Autodesk Inventor part; units mm, degrees
(part 2 of 2)
  spline S62 degree 3 poles (-7.4168, 223.4534) (-7.297, 223.2633) (-7.1172, 222.9781) (-6.8962, 222.5867) (-6.7374, 222.2894) (-6.5869, 221.9878) (-6.4451, 221.6819) (-6.3131, 221.3718) (-6.1917, 221.0573) (-6.0827, 220.7383) (-5.9867, 220.415) (-5.9243, 220.1411) (-5.8792, 219.921) (-5.8315, 219.7591) (-5.7671, 219.6031) (-5.6832, 219.4564) (-5.5947, 219.3467) (-5.5148, 219.2675) (-5.4472, 219.217) (-5.378, 219.1686) (-5.3017, 219.1325) (-5.2242, 219.099) (-5.1421, 219.0792) (-5.0594, 219.0625) (-4.9468, 219.0585) (-4.8065, 219.061) (-4.6661, 219.0585) (-4.5535, 219.0625) (-4.4708, 219.0792) (-4.3887, 219.099) (-4.3112, 219.1325) (-4.2349, 219.1686) (-4.1657, 219.217) (-4.0981, 219.2675) (-4.0182, 219.3467) (-3.9298, 219.4564) (-3.8458, 219.6031) (-3.7814, 219.7591) (-3.7338, 219.921) (-3.6887, 220.1411) (-3.6262, 220.415) (-3.5303, 220.7383) (-3.4212, 221.0573) (-3.2998, 221.3718) (-3.1678, 221.6819) (-3.0261, 221.9878) (-2.8756, 222.2894) (-2.7167, 222.5867) (-2.4957, 222.9781) (-2.3159, 223.2633) (-2.1961, 223.4534) knots -1.0784 -1.0784 -1.0784 -1.0784 -1.010995 -0.977291 -0.943586 -0.909882 -0.876178 -0.842474 -0.80877 -0.775067 -0.741365 -0.707665 -0.690816 -0.67397 -0.657123 -0.640284 -0.623449 -0.615023 -0.606598 -0.598176 -0.589749 -0.581327 -0.572901 -0.564477 -0.556053 -0.5392 -0.522347 -0.513923 -0.505499 -0.497074 -0.488651 -0.480225 -0.471802 -0.463377 -0.454951 -0.438116 -0.421277 -0.40443 -0.387584 -0.370735 -0.337035 -0.303333 -0.26963 -0.235926 -0.202222 -0.168518 -0.134814 -0.101109 -0.067405 0 0 0 0 construction
  line L30 (-2.1961, 223.4534) -> (-1.1338, 223.4534) construction
  spline S63 degree 3 poles (-1.1338, 223.4534) (-1.014, 223.2633) (-0.8342, 222.9781) (-0.6132, 222.5867) (-0.4544, 222.2894) (-0.3039, 221.9878) (-0.1621, 221.6819) (-0.0301, 221.3718) (0.0913, 221.0573) (0.2003, 220.7383) (0.2963, 220.415) (0.3587, 220.1411) (0.4038, 219.921) (0.4515, 219.7591) (0.5159, 219.6031) (0.5998, 219.4564) (0.6883, 219.3467) (0.7682, 219.2675) (0.8358, 219.217) (0.905, 219.1686) (0.9813, 219.1325) (1.0588, 219.099) (1.1409, 219.0792) (1.2236, 219.0625) (1.3362, 219.0585) (1.4765, 219.061) (1.6169, 219.0585) (1.7295, 219.0625) (1.8122, 219.0792) (1.8943, 219.099) (1.9718, 219.1325) (2.0481, 219.1686) (2.1173, 219.217) (2.1849, 219.2675) (2.2648, 219.3467) (2.3532, 219.4564) (2.4372, 219.6031) (2.5016, 219.7591) (2.5492, 219.921) (2.5943, 220.1411) (2.6568, 220.415) (2.7527, 220.7383) (2.8618, 221.0573) (2.9832, 221.3718) (3.1152, 221.6819) (3.2569, 221.9878) (3.4074, 222.2894) (3.5663, 222.5867) (3.7873, 222.9781) (3.9671, 223.2633) (4.0869, 223.4534) knots -1.0784 -1.0784 -1.0784 -1.0784 -1.010995 -0.977291 -0.943586 -0.909882 -0.876178 -0.842474 -0.80877 -0.775067 -0.741365 -0.707665 -0.690816 -0.67397 -0.657123 -0.640284 -0.623449 -0.615023 -0.606598 -0.598176 -0.589749 -0.581327 -0.572901 -0.564477 -0.556053 -0.5392 -0.522347 -0.513923 -0.505499 -0.497074 -0.488651 -0.480225 -0.471802 -0.463377 -0.454951 -0.438116 -0.421277 -0.40443 -0.387584 -0.370735 -0.337035 -0.303333 -0.26963 -0.235926 -0.202222 -0.168518 -0.134814 -0.101109 -0.067405 0 0 0 0 construction
  line L31 (4.0869, 223.4534) -> (5.1492, 223.4534) construction
  spline S64 degree 3 poles (5.1492, 223.4534) (5.269, 223.2633) (5.4488, 222.9781) (5.6698, 222.5867) (5.8286, 222.2894) (5.9791, 221.9878) (6.1209, 221.6819) (6.2529, 221.3718) (6.3743, 221.0573) (6.4833, 220.7383) (6.5793, 220.415) (6.6417, 220.1411) (6.6868, 219.921) (6.7345, 219.7591) (6.7989, 219.6031) (6.8828, 219.4564) (6.9713, 219.3467) (7.0512, 219.2675) (7.1188, 219.217) (7.188, 219.1686) (7.2643, 219.1325) (7.3418, 219.099) (7.4239, 219.0792) (7.5066, 219.0625) (7.6192, 219.0585) (7.7595, 219.061) (7.8999, 219.0585) (8.0125, 219.0625) (8.0952, 219.0792) (8.1773, 219.099) (8.2548, 219.1325) (8.3311, 219.1686) (8.4003, 219.217) (8.4679, 219.2675) (8.5478, 219.3467) (8.6362, 219.4564) (8.7202, 219.6031) (8.7846, 219.7591) (8.8322, 219.921) (8.8773, 220.1411) (8.9398, 220.415) (9.0357, 220.7383) (9.1448, 221.0573) (9.2662, 221.3718) (9.3982, 221.6819) (9.5399, 221.9878) (9.6904, 222.2894) (9.8493, 222.5867) (10.0703, 222.9781) (10.2501, 223.2633) (10.3699, 223.4534) knots -1.0784 -1.0784 -1.0784 -1.0784 -1.010995 -0.977291 -0.943586 -0.909882 -0.876178 -0.842474 -0.80877 -0.775067 -0.741365 -0.707665 -0.690816 -0.67397 -0.657123 -0.640284 -0.623449 -0.615023 -0.606598 -0.598176 -0.589749 -0.581327 -0.572901 -0.564477 -0.556053 -0.5392 -0.522347 -0.513923 -0.505499 -0.497074 -0.488651 -0.480225 -0.471802 -0.463377 -0.454951 -0.438116 -0.421277 -0.40443 -0.387584 -0.370735 -0.337035 -0.303333 -0.26963 -0.235926 -0.202222 -0.168518 -0.134814 -0.101109 -0.067405 0 0 0 0 construction
  line L32 (10.3699, 223.4534) -> (11.4322, 223.4534) construction
  spline S65 degree 3 poles (11.4322, 223.4534) (11.552, 223.2633) (11.7318, 222.9781) (11.9528, 222.5867) (12.1116, 222.2894) (12.2621, 221.9878) (12.4039, 221.6819) (12.5359, 221.3718) (12.6573, 221.0573) (12.7663, 220.7383) (12.8623, 220.415) (12.9247, 220.1411) (12.9698, 219.921) (13.0175, 219.7591) (13.0819, 219.6031) (13.1658, 219.4564) (13.2543, 219.3467) (13.3342, 219.2675) (13.4018, 219.217) (13.471, 219.1686) (13.5473, 219.1325) (13.6248, 219.099) (13.7069, 219.0792) (13.7896, 219.0625) (13.9022, 219.0585) (14.0425, 219.061) (14.1829, 219.0585) (14.2955, 219.0625) (14.3782, 219.0792) (14.4603, 219.099) (14.5378, 219.1325) (14.6141, 219.1686) (14.6833, 219.217) (14.7509, 219.2675) (14.8308, 219.3467) (14.9192, 219.4564) (15.0032, 219.6031) (15.0676, 219.7591) (15.1152, 219.921) (15.1603, 220.1411) (15.2228, 220.415) (15.3187, 220.7383) (15.4278, 221.0573) (15.5492, 221.3718) (15.6812, 221.6819) (15.8229, 221.9878) (15.9734, 222.2894) (16.1323, 222.5867) (16.3533, 222.9781) (16.5331, 223.2633) (16.6529, 223.4534) knots -1.0784 -1.0784 -1.0784 -1.0784 -1.010995 -0.977291 -0.943586 -0.909882 -0.876178 -0.842474 -0.80877 -0.775067 -0.741365 -0.707665 -0.690816 -0.67397 -0.657123 -0.640284 -0.623449 -0.615023 -0.606598 -0.598176 -0.589749 -0.581327 -0.572901 -0.564477 -0.556053 -0.5392 -0.522347 -0.513923 -0.505499 -0.497074 -0.488651 -0.480225 -0.471802 -0.463377 -0.454951 -0.438116 -0.421277 -0.40443 -0.387584 -0.370735 -0.337035 -0.303333 -0.26963 -0.235926 -0.202222 -0.168518 -0.134814 -0.101109 -0.067405 0 0 0 0 construction
  line L33 (16.6529, 223.4534) -> (17.7152, 223.4534) construction
  spline S66 degree 3 poles (17.7152, 223.4534) (17.835, 223.2633) (18.0148, 222.9781) (18.2358, 222.5867) (18.3946, 222.2894) (18.5451, 221.9878) (18.6869, 221.6819) (18.8189, 221.3718) (18.9403, 221.0573) (19.0493, 220.7383) (19.1453, 220.415) (19.2077, 220.1411) (19.2528, 219.921) (19.3005, 219.7591) (19.3649, 219.6031) (19.4488, 219.4564) (19.5373, 219.3467) (19.6172, 219.2675) (19.6848, 219.217) (19.754, 219.1686) (19.8303, 219.1325) (19.9078, 219.099) (19.9899, 219.0792) (20.0726, 219.0625) (20.1852, 219.0585) (20.3255, 219.061) (20.4659, 219.0585) (20.5785, 219.0625) (20.6612, 219.0792) (20.7433, 219.099) (20.8208, 219.1325) (20.8971, 219.1686) (20.9663, 219.217) (21.0339, 219.2675) (21.1138, 219.3467) (21.2022, 219.4564) (21.2862, 219.6031) (21.3506, 219.7591) (21.3982, 219.921) (21.4433, 220.1411) (21.5058, 220.415) (21.6017, 220.7383) (21.7108, 221.0573) (21.8322, 221.3718) (21.9642, 221.6819) (22.1059, 221.9878) (22.2564, 222.2894) (22.4153, 222.5867) (22.6363, 222.9781) (22.8161, 223.2633) (22.9359, 223.4534) knots -1.0784 -1.0784 -1.0784 -1.0784 -1.010995 -0.977291 -0.943586 -0.909882 -0.876178 -0.842474 -0.80877 -0.775067 -0.741365 -0.707665 -0.690816 -0.67397 -0.657123 -0.640284 -0.623449 -0.615023 -0.606598 -0.598176 -0.589749 -0.581327 -0.572901 -0.564477 -0.556053 -0.5392 -0.522347 -0.513923 -0.505499 -0.497074 -0.488651 -0.480225 -0.471802 -0.463377 -0.454951 -0.438116 -0.421277 -0.40443 -0.387584 -0.370735 -0.337035 -0.303333 -0.26963 -0.235926 -0.202222 -0.168518 -0.134814 -0.101109 -0.067405 0 0 0 0 construction
  line L34 (22.9359, 223.4534) -> (23.9982, 223.4534) construction
  spline S67 degree 3 poles (23.9982, 223.4534) (24.118, 223.2633) (24.2978, 222.9781) (24.5188, 222.5867) (24.6776, 222.2894) (24.8281, 221.9878) (24.9699, 221.6819) (25.1019, 221.3718) (25.2233, 221.0573) (25.3323, 220.7383) (25.4283, 220.415) (25.4907, 220.1411) (25.5358, 219.921) (25.5835, 219.7591) (25.6479, 219.6031) (25.7318, 219.4564) (25.8203, 219.3467) (25.9002, 219.2675) (25.9678, 219.217) (26.037, 219.1686) (26.1133, 219.1325) (26.1908, 219.099) (26.2729, 219.0792) (26.3556, 219.0625) (26.4682, 219.0585) (26.6085, 219.061) (26.7489, 219.0585) (26.8615, 219.0625) (26.9442, 219.0792) (27.0263, 219.099) (27.1038, 219.1325) (27.1801, 219.1686) (27.2493, 219.217) (27.3169, 219.2675) (27.3968, 219.3467) (27.4852, 219.4564) (27.5692, 219.6031) (27.6336, 219.7591) (27.6812, 219.921) (27.7263, 220.1411) (27.7888, 220.415) (27.8847, 220.7383) (27.9938, 221.0573) (28.1152, 221.3718) (28.2472, 221.6819) (28.3889, 221.9878) (28.5394, 222.2894) (28.6983, 222.5867) (28.9193, 222.9781) (29.0991, 223.2633) (29.2189, 223.4534) knots -1.0784 -1.0784 -1.0784 -1.0784 -1.010995 -0.977291 -0.943586 -0.909882 -0.876178 -0.842474 -0.80877 -0.775067 -0.741365 -0.707665 -0.690816 -0.67397 -0.657123 -0.640284 -0.623449 -0.615023 -0.606598 -0.598176 -0.589749 -0.581327 -0.572901 -0.564477 -0.556053 -0.5392 -0.522347 -0.513923 -0.505499 -0.497074 -0.488651 -0.480225 -0.471802 -0.463377 -0.454951 -0.438116 -0.421277 -0.40443 -0.387584 -0.370735 -0.337035 -0.303333 -0.26963 -0.235926 -0.202222 -0.168518 -0.134814 -0.101109 -0.067405 0 0 0 0 construction
  line L35 (29.2189, 223.4534) -> (30.2812, 223.4534) construction
  spline S68 degree 3 poles (30.2812, 223.4534) (30.401, 223.2633) (30.5808, 222.9781) (30.8018, 222.5867) (30.9606, 222.2894) (31.1111, 221.9878) (31.2529, 221.6819) (31.3849, 221.3718) (31.5063, 221.0573) (31.6153, 220.7383) (31.7113, 220.415) (31.7737, 220.1411) (31.8188, 219.921) (31.8665, 219.7591) (31.9309, 219.6031) (32.0148, 219.4564) (32.1033, 219.3467) (32.1832, 219.2675) (32.2508, 219.217) (32.32, 219.1686) (32.3963, 219.1325) (32.4738, 219.099) (32.5559, 219.0792) (32.6386, 219.0625) (32.7512, 219.0585) (32.8915, 219.061) (33.0319, 219.0585) (33.1445, 219.0625) (33.2272, 219.0792) (33.3093, 219.099) (33.3868, 219.1325) (33.4631, 219.1686) (33.5323, 219.217) (33.5999, 219.2675) (33.6798, 219.3467) (33.7682, 219.4564) (33.8522, 219.6031) (33.9166, 219.7591) (33.9642, 219.921) (34.0093, 220.1411) (34.0718, 220.415) (34.1677, 220.7383) (34.2768, 221.0573) (34.3982, 221.3718) (34.5302, 221.6819) (34.6719, 221.9878) (34.8224, 222.2894) (34.9813, 222.5867) (35.2023, 222.9781) (35.3821, 223.2633) (35.5019, 223.4534) knots -1.0784 -1.0784 -1.0784 -1.0784 -1.010995 -0.977291 -0.943586 -0.909882 -0.876178 -0.842474 -0.80877 -0.775067 -0.741365 -0.707665 -0.690816 -0.67397 -0.657123 -0.640284 -0.623449 -0.615023 -0.606598 -0.598176 -0.589749 -0.581327 -0.572901 -0.564477 -0.556053 -0.5392 -0.522347 -0.513923 -0.505499 -0.497074 -0.488651 -0.480225 -0.471802 -0.463377 -0.454951 -0.438116 -0.421277 -0.40443 -0.387584 -0.370735 -0.337035 -0.303333 -0.26963 -0.235926 -0.202222 -0.168518 -0.134814 -0.101109 -0.067405 0 0 0 0 construction
  line L36 (35.5019, 223.4534) -> (36.5642, 223.4534) construction
  spline S69 degree 3 poles (36.5642, 223.4534) (36.684, 223.2633) (36.8638, 222.9781) (37.0848, 222.5867) (37.2436, 222.2894) (37.3941, 221.9878) (37.5359, 221.6819) (37.6679, 221.3718) (37.7893, 221.0573) (37.8983, 220.7383) (37.9943, 220.415) (38.0567, 220.1411) (38.1018, 219.921) (38.1495, 219.7591) (38.2139, 219.6031) (38.2978, 219.4564) (38.3863, 219.3467) (38.4662, 219.2675) (38.5338, 219.217) (38.603, 219.1686) (38.6793, 219.1325) (38.7568, 219.099) (38.8389, 219.0792) (38.9216, 219.0625) (39.0342, 219.0585) (39.1745, 219.061) (39.3149, 219.0585) (39.4275, 219.0625) (39.5102, 219.0792) (39.5923, 219.099) (39.6698, 219.1325) (39.7461, 219.1686) (39.8153, 219.217) (39.8829, 219.2675) (39.9628, 219.3467) (40.0512, 219.4564) (40.1352, 219.6031) (40.1996, 219.7591) (40.2472, 219.921) (40.2923, 220.1411) (40.3548, 220.415) (40.4507, 220.7383) (40.5598, 221.0573) (40.6812, 221.3718) (40.8132, 221.6819) (40.9549, 221.9878) (41.1054, 222.2894) (41.2643, 222.5867) (41.4853, 222.9781) (41.6651, 223.2633) (41.7849, 223.4534) knots -1.0784 -1.0784 -1.0784 -1.0784 -1.010995 -0.977291 -0.943586 -0.909882 -0.876178 -0.842474 -0.80877 -0.775067 -0.741365 -0.707665 -0.690816 -0.67397 -0.657123 -0.640284 -0.623449 -0.615023 -0.606598 -0.598176 -0.589749 -0.581327 -0.572901 -0.564477 -0.556053 -0.5392 -0.522347 -0.513923 -0.505499 -0.497074 -0.488651 -0.480225 -0.471802 -0.463377 -0.454951 -0.438116 -0.421277 -0.40443 -0.387584 -0.370735 -0.337035 -0.303333 -0.26963 -0.235926 -0.202222 -0.168518 -0.134814 -0.101109 -0.067405 0 0 0 0 construction
  line L37 (41.7849, 223.4534) -> (42.8472, 223.4534) construction
  spline S70 degree 3 poles (42.8472, 223.4534) (42.967, 223.2633) (43.1468, 222.9781) (43.3678, 222.5867) (43.5266, 222.2894) (43.6771, 221.9878) (43.8189, 221.6819) (43.9509, 221.3718) (44.0723, 221.0573) (44.1813, 220.7383) (44.2773, 220.415) (44.3397, 220.1411) (44.3848, 219.921) (44.4325, 219.7591) (44.4969, 219.6031) (44.5808, 219.4564) (44.6693, 219.3467) (44.7492, 219.2675) (44.8168, 219.217) (44.886, 219.1686) (44.9623, 219.1325) (45.0398, 219.099) (45.1219, 219.0792) (45.2046, 219.0625) (45.3172, 219.0585) (45.4575, 219.061) (45.5979, 219.0585) (45.7105, 219.0625) (45.7932, 219.0792) (45.8753, 219.099) (45.9528, 219.1325) (46.0291, 219.1686) (46.0983, 219.217) (46.1659, 219.2675) (46.2458, 219.3467) (46.3342, 219.4564) (46.4182, 219.6031) (46.4826, 219.7591) (46.5302, 219.921) (46.5753, 220.1411) (46.6378, 220.415) (46.7337, 220.7383) (46.8428, 221.0573) (46.9642, 221.3718) (47.0962, 221.6819) (47.2379, 221.9878) (47.3884, 222.2894) (47.5473, 222.5867) (47.7683, 222.9781) (47.9481, 223.2633) (48.0679, 223.4534) knots -1.0784 -1.0784 -1.0784 -1.0784 -1.010995 -0.977291 -0.943586 -0.909882 -0.876178 -0.842474 -0.80877 -0.775067 -0.741365 -0.707665 -0.690816 -0.67397 -0.657123 -0.640284 -0.623449 -0.615023 -0.606598 -0.598176 -0.589749 -0.581327 -0.572901 -0.564477 -0.556053 -0.5392 -0.522347 -0.513923 -0.505499 -0.497074 -0.488651 -0.480225 -0.471802 -0.463377 -0.454951 -0.438116 -0.421277 -0.40443 -0.387584 -0.370735 -0.337035 -0.303333 -0.26963 -0.235926 -0.202222 -0.168518 -0.134814 -0.101109 -0.067405 0 0 0 0 construction
  line L38 (48.0679, 223.4534) -> (49.1302, 223.4534) construction
  spline S71 degree 3 poles (49.1302, 223.4534) (49.25, 223.2633) (49.4298, 222.9781) (49.6508, 222.5867) (49.8096, 222.2894) (49.9601, 221.9878) (50.1019, 221.6819) (50.2339, 221.3718) (50.3553, 221.0573) (50.4643, 220.7383) (50.5603, 220.415) (50.6227, 220.1411) (50.6678, 219.921) (50.7155, 219.7591) (50.7799, 219.6031) (50.8638, 219.4564) (50.9523, 219.3467) (51.0322, 219.2675) (51.0998, 219.217) (51.169, 219.1686) (51.2453, 219.1325) (51.3228, 219.099) (51.4049, 219.0792) (51.4876, 219.0625) (51.6002, 219.0585) (51.7405, 219.061) (51.8809, 219.0585) (51.9935, 219.0625) (52.0762, 219.0792) (52.1583, 219.099) (52.2358, 219.1325) (52.3121, 219.1686) (52.3813, 219.217) (52.4489, 219.2675) (52.5288, 219.3467) (52.6172, 219.4564) (52.7012, 219.6031) (52.7656, 219.7591) (52.8132, 219.921) (52.8583, 220.1411) (52.9208, 220.415) (53.0167, 220.7383) (53.1258, 221.0573) (53.2472, 221.3718) (53.3792, 221.6819) (53.5209, 221.9878) (53.6714, 222.2894) (53.8303, 222.5867) (54.0513, 222.9781) (54.2311, 223.2633) (54.3509, 223.4534) knots -1.0784 -1.0784 -1.0784 -1.0784 -1.010995 -0.977291 -0.943586 -0.909882 -0.876178 -0.842474 -0.80877 -0.775067 -0.741365 -0.707665 -0.690816 -0.67397 -0.657123 -0.640284 -0.623449 -0.615023 -0.606598 -0.598176 -0.589749 -0.581327 -0.572901 -0.564477 -0.556053 -0.5392 -0.522347 -0.513923 -0.505499 -0.497074 -0.488651 -0.480225 -0.471802 -0.463377 -0.454951 -0.438116 -0.421277 -0.40443 -0.387584 -0.370735 -0.337035 -0.303333 -0.26963 -0.235926 -0.202222 -0.168518 -0.134814 -0.101109 -0.067405 0 0 0 0 construction
  line L39 (54.3509, 223.4534) -> (55.4132, 223.4534) construction
  spline S72 degree 3 poles (55.4132, 223.4534) (55.533, 223.2633) (55.7128, 222.9781) (55.9338, 222.5867) (56.0926, 222.2894) (56.2431, 221.9878) (56.3849, 221.6819) (56.5169, 221.3718) (56.6383, 221.0573) (56.7473, 220.7383) (56.8433, 220.415) (56.9057, 220.1411) (56.9508, 219.921) (56.9985, 219.7591) (57.0629, 219.6031) (57.1468, 219.4564) (57.2353, 219.3467) (57.3152, 219.2675) (57.3828, 219.217) (57.452, 219.1686) (57.5283, 219.1325) (57.6058, 219.099) (57.6879, 219.0792) (57.7706, 219.0625) (57.8832, 219.0585) (58.0235, 219.061) (58.1639, 219.0585) (58.2765, 219.0625) (58.3592, 219.0792) (58.4413, 219.099) (58.5188, 219.1325) (58.5951, 219.1686) (58.6643, 219.217) (58.7319, 219.2675) (58.8118, 219.3467) (58.9002, 219.4564) (58.9842, 219.6031) (59.0486, 219.7591) (59.0962, 219.921) (59.1413, 220.1411) (59.2038, 220.415) (59.2997, 220.7383) (59.4088, 221.0573) (59.5302, 221.3718) (59.6622, 221.6819) (59.8039, 221.9878) (59.9544, 222.2894) (60.1133, 222.5867) (60.3343, 222.9781) (60.5141, 223.2633) (60.6339, 223.4534) knots -1.0784 -1.0784 -1.0784 -1.0784 -1.010995 -0.977291 -0.943586 -0.909882 -0.876178 -0.842474 -0.80877 -0.775067 -0.741365 -0.707665 -0.690816 -0.67397 -0.657123 -0.640284 -0.623449 -0.615023 -0.606598 -0.598176 -0.589749 -0.581327 -0.572901 -0.564477 -0.556053 -0.5392 -0.522347 -0.513923 -0.505499 -0.497074 -0.488651 -0.480225 -0.471802 -0.463377 -0.454951 -0.438116 -0.421277 -0.40443 -0.387584 -0.370735 -0.337035 -0.303333 -0.26963 -0.235926 -0.202222 -0.168518 -0.134814 -0.101109 -0.067405 0 0 0 0 construction
  line L40 (60.6339, 223.4534) -> (61.6962, 223.4534) construction
  spline S73 degree 3 poles (61.6962, 223.4534) (61.816, 223.2633) (61.9958, 222.9781) (62.2168, 222.5867) (62.3756, 222.2894) (62.5261, 221.9878) (62.6679, 221.6819) (62.7999, 221.3718) (62.9213, 221.0573) (63.0303, 220.7383) (63.1263, 220.415) (63.1887, 220.1411) (63.2338, 219.921) (63.2815, 219.7591) (63.3459, 219.6031) (63.4298, 219.4564) (63.5183, 219.3467) (63.5982, 219.2675) (63.6658, 219.217) (63.735, 219.1686) (63.8113, 219.1325) (63.8888, 219.099) (63.9709, 219.0792) (64.0536, 219.0625) (64.1662, 219.0585) (64.3065, 219.061) (64.4469, 219.0585) (64.5595, 219.0625) (64.6422, 219.0792) (64.7243, 219.099) (64.8018, 219.1325) (64.8781, 219.1686) (64.9473, 219.217) (65.0149, 219.2675) (65.0948, 219.3467) (65.1832, 219.4564) (65.2672, 219.6031) (65.3316, 219.7591) (65.3792, 219.921) (65.4243, 220.1411) (65.4868, 220.415) (65.5827, 220.7383) (65.6918, 221.0573) (65.8132, 221.3718) (65.9452, 221.6819) (66.0869, 221.9878) (66.2374, 222.2894) (66.3963, 222.5867) (66.6173, 222.9781) (66.7971, 223.2633) (66.9169, 223.4534) knots -1.0784 -1.0784 -1.0784 -1.0784 -1.010995 -0.977291 -0.943586 -0.909882 -0.876178 -0.842474 -0.80877 -0.775067 -0.741365 -0.707665 -0.690816 -0.67397 -0.657123 -0.640284 -0.623449 -0.615023 -0.606598 -0.598176 -0.589749 -0.581327 -0.572901 -0.564477 -0.556053 -0.5392 -0.522347 -0.513923 -0.505499 -0.497074 -0.488651 -0.480225 -0.471802 -0.463377 -0.454951 -0.438116 -0.421277 -0.40443 -0.387584 -0.370735 -0.337035 -0.303333 -0.26963 -0.235926 -0.202222 -0.168518 -0.134814 -0.101109 -0.067405 0 0 0 0 construction
  line L41 (66.9169, 223.4534) -> (67.9792, 223.4534) construction
  spline S74 degree 3 poles (67.9792, 223.4534) (68.099, 223.2633) (68.2788, 222.9781) (68.4998, 222.5867) (68.6586, 222.2894) (68.8091, 221.9878) (68.9509, 221.6819) (69.0829, 221.3718) (69.2043, 221.0573) (69.3133, 220.7383) (69.4093, 220.415) (69.4717, 220.1411) (69.5168, 219.921) (69.5645, 219.7591) (69.6289, 219.6031) (69.7128, 219.4564) (69.8013, 219.3467) (69.8812, 219.2675) (69.9488, 219.217) (70.018, 219.1686) (70.0943, 219.1325) (70.1718, 219.099) (70.2539, 219.0792) (70.3366, 219.0625) (70.4492, 219.0585) (70.5895, 219.061) (70.7299, 219.0585) (70.8425, 219.0625) (70.9252, 219.0792) (71.0073, 219.099) (71.0848, 219.1325) (71.1611, 219.1686) (71.2303, 219.217) (71.2979, 219.2675) (71.3778, 219.3467) (71.4662, 219.4564) (71.5502, 219.6031) (71.6146, 219.7591) (71.6622, 219.921) (71.7073, 220.1411) (71.7698, 220.415) (71.8657, 220.7383) (71.9748, 221.0573) (72.0962, 221.3718) (72.2282, 221.6819) (72.3699, 221.9878) (72.5204, 222.2894) (72.6793, 222.5867) (72.9003, 222.9781) (73.0801, 223.2633) (73.1999, 223.4534) knots -1.0784 -1.0784 -1.0784 -1.0784 -1.010995 -0.977291 -0.943586 -0.909882 -0.876178 -0.842474 -0.80877 -0.775067 -0.741365 -0.707665 -0.690816 -0.67397 -0.657123 -0.640284 -0.623449 -0.615023 -0.606598 -0.598176 -0.589749 -0.581327 -0.572901 -0.564477 -0.556053 -0.5392 -0.522347 -0.513923 -0.505499 -0.497074 -0.488651 -0.480225 -0.471802 -0.463377 -0.454951 -0.438116 -0.421277 -0.40443 -0.387584 -0.370735 -0.337035 -0.303333 -0.26963 -0.235926 -0.202222 -0.168518 -0.134814 -0.101109 -0.067405 0 0 0 0 construction
  line L42 (73.1999, 223.4534) -> (74.2622, 223.4534) construction
  spline S75 degree 3 poles (74.2622, 223.4534) (74.5153, 223.0519) (75.0923, 222.1366) (75.8167, 220.1456) (75.7693, 219.7983) (76.0967, 219.3157) (76.2034, 219.2355) (76.307, 219.166) (76.4035, 219.106) (76.6971, 219.0474) (76.833, 219.0601) (77.0832, 219.0592) (77.1939, 219.0617) (77.418, 219.1519) (77.5117, 219.2124) (77.6509, 219.3283) (77.7123, 219.4106) (77.8212, 219.569) (77.8771, 219.6969) (77.9737, 220.0135) (77.9892, 220.1745) (78.4659, 221.8916) (79.3072, 223.1746) (79.4829, 223.4534) knots 0 0 0 0 0.142394 0.142394 0.262557 0.262557 0.314666 0.314666 0.34653 0.34653 0.372217 0.372217 0.394622 0.394622 0.411062 0.411062 0.432958 0.432958 0.48678 0.48678 0.562983 0.562983 0.900876 0.900876 0.900876 0.900876 construction
  line L43 (79.4829, 223.4534) -> (79.4829, 214.06) construction
  line L44 (79.4829, 214.06) -> (-20.5171, 214.06) construction
  line L45 (-20.5171, 214.06) -> (-20.5171, 223.4534) construction
  line L46 (-20.5171, 223.4534) -> (-19.9828, 223.4534) construction
  line L47 (64.2812, 213.91) -> (6.11, 213.91)
  line L48 (64.2812, 256.0593) -> (54.2812, 256.0593)
  line L49 (54.2812, 256.0593) -> (54.2812, 246.0593)
  line L50 (54.2812, 246.0593) -> (64.2812, 246.0593)
  line L51 (64.2812, 246.0593) -> (64.2812, 256.0593)
  line L52 (6.1102, 256.0593) -> (6.1102, 246.0593)
  line L53 (6.1102, 246.0593) -> (16.1102, 246.0593)
  line L54 (16.1102, 256.0593) -> (6.1102, 256.0593)
  line L55 (16.1102, 246.0593) -> (16.1102, 256.0593)
  line L56 (54.2812, 213.9103) -> (54.2812, 203.9103)
  line L57 (54.2812, 203.9103) -> (64.2812, 203.9103)
  line L58 (64.2812, 213.9103) -> (54.2812, 213.9103)
  line L59 (64.2812, 203.9103) -> (64.2812, 213.9103)
  line L60 (6.1102, 213.9103) -> (6.1102, 203.9103)
  line L61 (6.1102, 203.9103) -> (16.1102, 203.9103)
  line L62 (16.1102, 213.9103) -> (6.1102, 213.9103)
  line L63 (16.1102, 203.9103) -> (16.1102, 213.9103)
  circle A38 centre (59.2812, 251.0593) radius 1.25
  circle A39 centre (59.2812, 208.9103) radius 1.25
  circle A40 centre (11.1102, 251.0593) radius 1.25
  circle A41 centre (11.1102, 208.9103) radius 1.25
  point P0 (64.2812, 0)
  point P1 (6.11, 256.0593)
  dimension "d0" = 10.15
  dimension "d1" = 0.15
  dimension "d2" = 12
  dimension "d3" = 10
  dimension "d4" = 10
  dimension "d7" = 48.171
  dimension "d10" = 42.149
  dimension "d13" = 2.5
  dimension "d16" = 42.149
  dimension "d19" = 48.171
  constraints: 42 end point, 4 centre point, 4 horizontal, 4 parallel, 4 point on line, 3 perpendicular, 2 vertical, 30 other
  measures "d0" distance between parallel lines of L44 L10
  measures "d1" distance between parallel lines of L44 L47
  measures "d2" distance from line of A37.end L8
  measures "d3" distance of L50.end L49.end
  measures "d4" distance of L49.end L48.end
  measures "d7" distance of L48.end L52.start
  measures "d10" distance of L48.end L56.start
  measures "d13" diameter of A38
  measures "d16" distance of A38.centre A39.centre
  measures "d19" distance of A38.centre A40.centre
extrude "Extrusion1" add sketch "Sketch1" along normal blind 5 and the other way blind 5 contours L10 L56 L47 L0 | L47 L6 L53 L55 L8 L49 L50 L0 | L10 L63 L47 L56 | L6 L47 L63 L10 | L50 L49 L8 L0 | L6 L8 L55 L53
sketch "Sketch2" plane through (-58.1712, -256.0593, 13.749) normal (0, -1, 0) x (1, 0, 0)
  line L0 (58.1712, 4.271) -> (56.0979, 4.271) projected
  arc A0 (56.0979, 4.271) -> (48.1592, 4.9999) centre (47.5772, -44.9369) ccw projected
  line L1 (48.1592, 4.9999) -> (48.1592, 4.0806) projected
  line L2 (48.1592, 4.0806) -> (46.2813, 4.0806) projected
  arc A1 (46.2813, 4.0806) -> (40.6924, 4.5096) centre (41.5081, -21.4831) ccw projected
  arc A2 (40.6924, 4.5096) -> (32.7872, 3.2449) centre (40.2264, -17.9175) ccw projected
  arc A3 (22.1478, 3.0708) -> (32.7872, 3.2449) centre (27.1272, 23.9496) ccw projected
  line L3 (22.1478, 3.0708) -> (20.1773, 3.0708) projected
  line L4 (20.1773, 3.0708) -> (20.1773, 1.9061) projected
  line L5 (20.1773, 1.9061) -> (16.4523, 1.9061) projected
  arc A4 (16.4523, 1.9061) -> (8.2145, 2.1113) centre (11.783, -20.0814) ccw projected
  arc A5 (6.4215, 2.2317) -> (8.2145, 2.1113) centre (7.6247, 6.7426) ccw projected
  line L6 (6.4215, 2.2317) -> (6.4215, 2.5959) projected
  arc A6 (6.4215, 2.5959) -> (1.9312, 2.1372) centre (9.2045, -46.8579) ccw projected
  line L7 (1.9312, 2.1372) -> (0, 2.2668) projected
  line L8 (0, 2.2668) -> (0, -4.8132) projected
  line L9 (0, -4.8132) -> (-6.11, -4.8132) projected
  line L10 (-6.11, -4.8132) -> (-6.11, -13.749) projected
  line L11 (-6.11, -13.749) -> (58.1712, -13.749) projected
  line L12 (58.1712, -13.749) -> (58.1712, 4.271) projected
  line L13 (58.1712, 0) -> (0, 0) projected
  line L14 (58.1712, 0) -> (-0.1521, 0)
  constraints: 2 end point, 1 collinear
extrude "Extrusion2" cut sketch "Sketch2" against normal through all contours L12 L13 L8 L7 A6 L6 A5 A4 L5 L4 L3 A3 A2 A1 L2 L1 A0 L0
body "Solid1"
